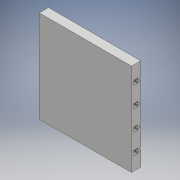
# Autodesk Inventor part: T-SLOT TABLE
Saved by Autodesk Inventor 2018 (Build 220112000, 112)
## iProperties
Created: 2018-10-13
Part Number: T-SLOT TABLE
Material: Generic
Document SubType Name: Modeling
Designer: Matthew Morey
Density: 1 g/cm^3
Appearance: Default
Author: Matthew Morey
Autodesk Inventor part; units mm, degrees
ref_plane "YZ Plane" through (0, 0, 0) normal (1, 0, 0) x (0, 1, 0)
ref_plane "XZ Plane" through (0, 0, 0) normal (0, 1, 0) x (-1, 0, 0)
ref_plane "XY Plane" through (0, 0, 0) normal (0, 0, 1) x (1, 0, 0)
sketch "Sketch1" plane through (0, 0, 0) normal (1, 0, 0) x (0, 1, 0)
  line L0 (0, 100) -> (0, -100)
  line L1 (0, 100) -> (20, 100)
  line L2 (20, 100) -> (20, 68)
  line L3 (20, 68) -> (13.5, 68)
  line L4 (13.5, 68) -> (13.5, 71)
  line L5 (13.5, 71) -> (5.5, 71)
  line L6 (5.5, 71) -> (5.5, 61)
  line L7 (5.5, 61) -> (13.5, 61)
  line L8 (13.5, 61) -> (13.5, 64)
  line L9 (13.5, 64) -> (20, 64)
  line L10 (20, 64) -> (20, 24)
  line L11 (20, 24) -> (13.5, 24)
  line L12 (13.5, 24) -> (13.5, 27)
  line L13 (13.5, 27) -> (5.5, 27)
  line L14 (5.5, 27) -> (5.5, 17)
  line L15 (5.5, 17) -> (13.5, 17)
  line L16 (13.5, 17) -> (13.5, 20)
  line L17 (13.5, 20) -> (20, 20)
  line L18 (20, 20) -> (20, -20)
  line L19 (20, -20) -> (13.5, -20)
  line L20 (13.5, -20) -> (13.5, -17)
  line L21 (13.5, -17) -> (5.5, -17)
  line L22 (5.5, -17) -> (5.5, -27)
  line L23 (5.5, -27) -> (13.5, -27)
  line L24 (13.5, -27) -> (13.5, -24)
  line L25 (13.5, -24) -> (20, -24)
  line L26 (20, -24) -> (20, -64)
  line L27 (20, -64) -> (13.5, -64)
  line L28 (13.5, -64) -> (13.5, -61)
  line L29 (13.5, -61) -> (5.5, -61)
  line L30 (5.5, -61) -> (5.5, -71)
  line L31 (5.5, -71) -> (13.5, -71)
  line L32 (13.5, -71) -> (13.5, -68)
  line L33 (13.5, -68) -> (20, -68)
  line L34 (20, -68) -> (20, -100)
  line L35 (0, -100) -> (20, -100)
  point P0 (0, 0)
  dimension "d0" = 200
  dimension "d1" = 100
  dimension "d2" = 20
  dimension "d3" = 32
  dimension "d4" = 6.5
  dimension "d5" = 3
  dimension "d6" = 8
  dimension "d7" = 10
  dimension "d8" = 8
  dimension "d9" = 3
  dimension "d10" = 6.5
  dimension "d11" = 40
  dimension "d12" = 6.5
  dimension "d13" = 3
  dimension "d14" = 8
  dimension "d15" = 10
  dimension "d16" = 8
  dimension "d17" = 3
  dimension "d18" = 6.5
  dimension "d19" = 40
  dimension "d20" = 6.5
  dimension "d21" = 3
  dimension "d22" = 8
  dimension "d23" = 10
  dimension "d24" = 8
  dimension "d25" = 3
  dimension "d26" = 6.5
  dimension "d27" = 40
  dimension "d28" = 6.5
  dimension "d29" = 3
  dimension "d30" = 8
  dimension "d31" = 10
  dimension "d32" = 8
  dimension "d33" = 3
  dimension "d34" = 6.5
  dimension "d35" = 32
  dimension "d36" = 20
  dimension "d37" = 7
  dimension "d38" = 83
  dimension "d39" = 34
  dimension "d40" = 142
  dimension "d41" = 20
  dimension "d42" = 17
  dimension "d43" = 20
  dimension "d44" = 24
  constraints: 72 end point, 26 point on line, 5 perpendicular, 3 horizontal, 1 parallel, 1 vertical
  measures "d0" distance of L0.start L0.end
  measures "d1" distance of L0.end point (0, 0)
  measures "d2" distance of L0.start L1.end
  measures "d3" distance of L1.end L2.end
  measures "d4" distance of L2.end L3.end
  measures "d5" distance of L3.end L4.end
  measures "d6" distance of L4.end L5.end
  measures "d7" distance of L5.end L6.end
  measures "d8" distance of L6.end L7.end
  measures "d9" distance of L7.end L8.end
  measures "d10" distance of L8.end L9.end
  measures "d11" distance of L9.end L10.end
  measures "d12" distance of L10.end L11.end
  measures "d13" distance of L11.end L12.end
  measures "d14" distance of L12.end L13.end
  measures "d15" distance of L13.end L14.end
  measures "d16" distance of L14.end L15.end
  measures "d17" distance of L15.end L16.end
  measures "d18" distance of L16.end L17.end
  measures "d19" distance of L17.end L18.end
  measures "d20" distance of L18.end L19.end
  measures "d21" distance of L19.end L20.end
  measures "d22" distance of L20.end L21.end
  measures "d23" distance of L21.end L22.end
  measures "d24" distance of L22.end L23.end
  measures "d25" distance of L23.end L24.end
  measures "d26" distance of L24.end L25.end
  measures "d27" distance of L25.end L26.end
  measures "d28" distance of L26.end L27.end
  measures "d29" distance of L27.end L28.end
  measures "d30" distance of L28.end L29.end
  measures "d31" distance of L29.end L30.end
  measures "d32" distance of L30.end L31.end
  measures "d33" distance of L31.end L32.end
  measures "d34" distance of L32.end L33.end
  measures "d35" distance of L33.end L34.end
  measures "d36" distance of L0.end L34.end
  measures "d37" distance between parallel lines of L11 L15
  measures "d38" distance between parallel lines of L21 L35
  measures "d39" distance between parallel lines of L23 L29
  measures "d40" distance between parallel lines of L31 L5
  measures "d41" distance from line of point (0, 0) L18
  measures "d42" distance from line of point (0, 0) L15
  measures "d43" distance from line of point (0, 0) L17
  measures "d44" distance from line of point (0, 0) L25
extrude "Extrusion1" add sketch "Sketch1" along normal blind 200
body "Solid1"
